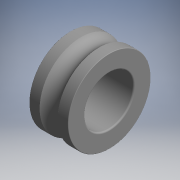
# Autodesk Inventor part: SKF_16100_PART1
Saved by Autodesk Inventor 2017.3 (Build 213256000, 256)
## iProperties
Part Number: SKF_16100_PART1
Material: Generic
Catalog Web Link: www.cadenas.de
Description: -Deep groove ball bearings
Vendor: SKF
Document SubType Name: Modeling
Designer: partserver
Manufacturer: SKF
Mass: 24 g
Surface Area: 9.76096 cm^2
Volume: 1.07006 cm^3
Density: 1 g/cm^3
Appearance: PSOLRGB-175-175-175
Category: PARTsolutions
Company: SKF
Title: SKF_16100_PART1
Author: Cadenas PARTsolutions
Comments: Deep groove ball bearings
PSOL_IDENT_0: {$CADENAS_DATA\23d-libs\skf\bearings_units_and_housings\ball_bearings\deep_groove_ball_bearings\bb1_
PSOL_IDENT_1: 001_101.prj},196 {VTYP=3D},{NB=SKF_16100_PART1},{LINA=SKF_16100_PART1},{NN=BB1_001_101_PART1},{NOPRJ=
PSOL_IDENT_2: TRUE},{DATE=18.06.2021 07:30:58},{GEOMDATE=16.06.2021 12:48:44},{VERSION=},{LINEID=5530},{WBVAR=},{W
PSOL_IDENT_3: BNUMERIC=}  {NB=SKF_16100_PART1},{LINA=SKF_16100_PART1},{KT=DUMMY},{DESIGNATION=16100},{R12=0.30},{D
PSOL_IDENT_4: D=10.000},{D=28.000},{B=8.000},{C=},{CX=},{CXX=},{CA=0.000},{XXVARIANT=},{XXDESIGN=Single row},{XXSE
PSOL_IDENT_5: ALING=No seals},{DESIGN=dgbb1},{DESIGNIR=dgbb1},{VARIANT=},{DD1=17.00},{DD2=},{DD2X=},{DD2A=0.00},{D
PSOL_IDENT_6: 1=23.20},{D1X=MIN},{D2=24.72},{D2A=24.72},{D3=},{D3X=},{D3A=0.000},{D4=},{HH=MIN},{BB=MIN},{BBX=},{B
PSOL_IDENT_7: BA=0.000},{FF=},{R0MAX=MIN},{R0=MIN},{PITCH=20.00},{DW=4.762},{DDAMIN=14.200},{DDAMAX=MIN},{DDBMIN=M
PSOL_IDENT_8: IN},{DDBMAX=MIN},{DBMIN=MIN},{DAMAX=23.800},{BBAMIN=MIN},{CAMAX=MIN},{RAMAX=0.300},{LOAD1=5.070},{LO
PSOL_IDENT_9: AD2=2.360},{LOAD3=0.100},{SPEED1=60000},{SPEED2=38000},{KR=0.025},{F0=13.100},{Z=8},{II=1},{MASS=0.0
PSOL_IDENT_10: 24},{BEARING=16100},{RING=},{HELP=2.400},{HELP2=1.640},{DD1ALG=8.500},{YALG=8.500},{PITCH1=20.000},{
PSOL_IDENT_11: DW1=4.762},{YALG1=11.600},{HALG1=2.400},{SH=8.500},{CU=0.648},{HALG=3.5},{B1=0},{SHIELDHELP=1},{D4A=
PSOL_IDENT_12: 0.000},{FFA=0.000},{RS1=}
NB: SKF_16100_PART1
NT: Deep groove ball bearings
NBSYN: SKF_$DESIGNATION._PART1
LINA: SKF_16100_PART1
CATALOG: SKF
DESIGNATION: 16100
R12: 0.3
DD: 10
D: 28
B: 8
D2: 24.72
LOAD1: 5.07
LOAD2: 2.36
LOAD3: 0.1
SPEED1: 60000
SPEED2: 38000
BEARING: 16100
SUPPLIER: SKF
ARTICLENO: SKF_16100_PART1
BOMINFO: SKF_16100_PART1
CREATOR: CADENAS GmbH
Autodesk Inventor part; units mm, degrees
ref_plane "YZ Plane" through (0, 0, 0) normal (1, 0, 0) x (0, 1, 0)
ref_plane "XZ Plane" through (0, 0, 0) normal (0, 1, 0) x (-1, 0, 0)
ref_plane "XY Plane" through (0, 0, 0) normal (0, 0, 1) x (1, 0, 0)
sketch "Sketch_54" plane through (0, 0, 0) normal (0, 0, 1) x (1, 0, 0)
  line L0 (100, 0) -> (-100, 0)
  arc A0 (0, 5.3) -> (0.3, 5) centre (0.3, 5.3) ccw
  line L1 (0.3, 5) -> (7.7, 5)
  arc A1 (7.7, 5) -> (8, 5.3) centre (7.7, 5.3) ccw
  line L2 (8, 5.3) -> (8, 8.4)
  arc A2 (8, 8.4) -> (7.9, 8.5) centre (7.9, 8.4) ccw
  line L3 (7.9, 8.5) -> (5.8491, 8.5)
  arc A3 (2.1509, 8.5) -> (5.8491, 8.5) centre (4, 10) ccw
  line L4 (2.1509, 8.5) -> (0.1, 8.5)
  arc A4 (0.1, 8.5) -> (0, 8.4) centre (0.1, 8.4) ccw
  line L5 (0, 8.4) -> (0, 5.3)
  constraints: 12 end point, 10 point on circle, 5 centre point
revolve "Revolution1" add sketch "Sketch_54" angle 360 about axis through (100, 0, 0) along (1, 0, 0)
body "Solid1"
